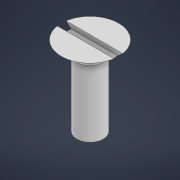
# Autodesk Inventor part: Pieza10 IG
Saved by Autodesk Inventor 2021 (Build 250183000, 183)
## iProperties
Created: 2020-10-13
Part Number: Pieza10 IG
Material: Generic
Document SubType Name: Modeling
Designer: iran1
Density: 1 g/cm^3
Appearance: Default
Author: iran1
Autodesk Inventor part; units mm, degrees
ref_plane "YZ Plane" through (0, 0, 0) normal (1, 0, 0) x (0, 1, 0)
ref_plane "XZ Plane" through (0, 0, 0) normal (0, 1, 0) x (-1, 0, 0)
ref_plane "XY Plane" through (0, 0, 0) normal (0, 0, 1) x (1, 0, 0)
sketch "Sketch1" plane through (0, 0, 0) normal (0, 0, 1) x (1, 0, 0)
  line L0 (0, 15.0207) -> (0, -34.9793) construction
  line L1 (0, 15.0207) -> (50, 15.0207) construction
  line L2 (0, 0) -> (1, 0)
  line L3 (1, 0) -> (1, 1)
  line L4 (1, 1) -> (6.5, 1)
  line L5 (6.5, 1) -> (3, -2)
  line L6 (3, -2) -> (3, -17)
  line L7 (3, -17) -> (0, -18.7321)
  line L8 (0, -26.021) -> (0, -26.021)
  line L9 (0, 0) -> (0, -18.7321)
  dimension "d4" = 50
  dimension "d6" = 1
  dimension "d7" = 1
  dimension "d8" = 5.5
  dimension "d9" = 3
  dimension "d10" = 0
  dimension "d11" = 0
  dimension "d12" = 15
  dimension "d13" = 3
  dimension "d15" = 60
  dimension "d17" = 60
  dimension "d18" = 139.399
  dimension "d19" = 15.0207
  dimension "d20" = 41.0417
  constraints: 20 end point, 3 perpendicular, 3 point on line, 2 horizontal, 1 collinear, 1 parallel, 1 vertical
  measures "d4" distance of L0.start L0.end
  measures "d6" distance of L2.start L2.end
  measures "d7" distance of L2.end L3.end
  measures "d8" distance of L3.end L4.end
  measures "d9" distance between parallel lines of L0 L6
  measures "d10" distance of point (0, 0) L2.start
  measures "d11" distance of point (0, 0) L2.start
  measures "d12" distance of L5.end L6.end
  measures "d13" distance from line of L4 L5.end
  measures "d15" angle of L8 L7
  measures "d17" angle of L0 L7
  measures "d18" angle of L5 L1
  measures "d19" distance between parallel lines of L2 L1
  measures "d20" distance from line of L8.end L1
revolve "Revolution1" add sketch "Sketch1" angle 360 about axis through (0, 15.0207, 0) along (0, -1, 0)
sketch "Sketch2" plane through (0, 1, 0) normal (0, 1, 0) x (1, 0, 0)
  line L0 (-12.6442, -1) -> (7.3558, -1)
  line L1 (7.3558, -1) -> (7.3558, 1)
  line L2 (7.3558, 1) -> (-12.6442, 1)
  line L3 (-12.6442, 1) -> (-12.6442, -1)
  circle A0 centre (0, 0) radius 1 projected
  dimension "d23" = 20
  dimension "d24" = 2
  dimension "d25" = 0
  constraints: 8 end point, 2 parallel, 1 horizontal, 1 perpendicular
  measures "d23" distance of L2.end L1.end
  measures "d24" distance of L1.end L0.end
  measures "d25" distance edge to line of A0 L2
extrude "Extrusion1" cut sketch "Sketch2" against normal blind 1
body "Solid1"
